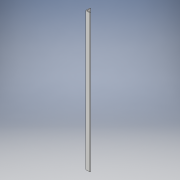
# Autodesk Inventor part: BumperMount1-ver1-1111-2019
Saved by Autodesk Inventor 2018 (Build 220112000, 112)
## iProperties
Created: 2020-01-11
Part Number: BumperMount1-ver1-1111-2019
Material: Generic
Document SubType Name: Modeling
Designer: JMHal
Density: 1 g/cm^3
Appearance: Default
Author: JMHal
Autodesk Inventor part; units mm, degrees
ref_plane "YZ Plane" through (0, 0, 0) normal (1, 0, 0) x (0, 1, 0)
ref_plane "XZ Plane" through (0, 0, 0) normal (0, 1, 0) x (-1, 0, 0)
ref_plane "XY Plane" through (0, 0, 0) normal (0, 0, 1) x (1, 0, 0)
sketch "Sketch3" plane through (0, 0, 0) normal (0, 1, 0) x (-1, 0, 0)
  line L0 (0, 0) -> (25.4, 0)
  line L1 (25.4, 0) -> (25.4, -3.175)
  line L2 (25.4, -3.175) -> (0, -3.175)
  line L3 (0, -3.175) -> (0, 0)
  line L4 (25.4, 0) -> (22.225, 0)
  line L5 (22.225, 0) -> (22.225, -25.4)
  line L6 (22.225, -25.4) -> (25.4, -25.4)
  line L7 (25.4, -25.4) -> (25.4, 0)
  dimension "d8" = 25.4
  dimension "d9" = 3.175
  dimension "d10" = 3.175
  dimension "d11" = 25.4
  constraints: 16 end point, 4 parallel, 2 horizontal, 2 perpendicular
  measures "d8" distance of L1.end L2.end
  measures "d9" distance between parallel lines of L2 L0
  measures "d10" distance between parallel lines of L5 L7
  measures "d11" distance between parallel lines of L6 L0
extrude "Extrusion3" add sketch "Sketch3" along normal blind 812.8
sketch "Sketch4" plane through (-25.4, 0, -25.4) normal (-1, 0, 0) x (0, 0, 1)
  circle A0 centre (9.525, 292.1) radius 2.0701
  line L0 (0, 0) -> (25.4, 0) projected
  line L1 (0, 0) -> (0, 812.8) projected
  line L2 (25.4, 0) -> (25.4, 812.8) projected
  dimension "d14" = 4.1402
  dimension "d15" = 292.1
  dimension "d21" = 9.525
  constraints: 1 centre point
  measures "d14" diameter of A0
  measures "d15" distance from line of A0.centre L0
  measures "d21" distance from line of A0.centre L1
extrude "Extrusion4" cut sketch "Sketch4" against normal blind 25.4
sketch "Sketch5" plane through (-25.4, 0, -25.4) normal (-1, 0, 0) x (0, 0, 1)
  circle A0 centre (9.525, 520.7) radius 2.0701
  line L0 (0, 0) -> (0, 812.8) projected
  circle A1 centre (9.525, 292.1) radius 2.0701 projected
  point P0 (25.4, 0)
  dimension "d25" = 4.1402
  dimension "d26" = 9.525
  dimension "d27" = 228.6
  constraints: 1 centre point
  measures "d25" diameter of A0
  measures "d26" distance from line of A0.centre L0
  measures "d27" distance of A1.centre A0.centre
extrude "Extrusion5" cut sketch "Sketch5" against normal blind 25.4 contours A0
sketch "Sketch6" plane through (-25.4, 0, -25.4) normal (-1, 0, 0) x (0, 0, 1)
  circle A0 centre (11.5951, 12.7) radius 2.0701
  line L0 (0, 0) -> (0, 812.8) projected
  circle A1 centre (9.525, 292.1) radius 2.0701 projected
  circle A2 centre (9.525, 800.1) radius 2.0701
  circle A3 centre (9.525, 520.7) radius 2.0701 projected
  point P0 (25.4, 0)
  dimension "d30" = 4.1402
  dimension "d31" = 9.525
  dimension "d32" = 279.4
  dimension "d33" = 4.1402
  dimension "d34" = 9.525
  dimension "d35" = 279.4
  constraints: 2 centre point
  measures "d30" diameter of A0
  measures "d31" distance edge to line of A0 L0
  measures "d32" vertical distance of A1.centre A0.centre
  measures "d33" diameter of A2
  measures "d34" distance from line of A2.centre L0
  measures "d35" distance of A3.centre A2.centre
extrude "Extrusion6" cut sketch "Sketch6" against normal blind 25.4 contours A0 | A2
body "Solid3"
